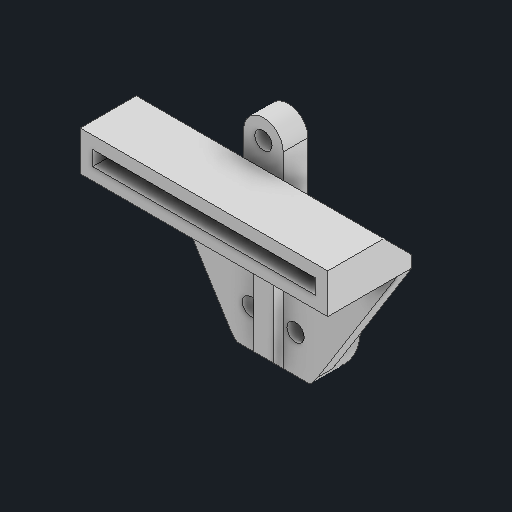
# Autodesk Inventor part: Lazercutlink
Saved by Autodesk Inventor 2026.1 (Build 301233000, 233)
## iProperties
Created: 2025-10-02
Part Number: Lazercutlink
Material: Generic
Document SubType Name: Modeling
Designer: Malthe Sennels
Density: 1 g/cm^3
Appearance: Default
Author: Malthe Sennels
Autodesk Inventor part; units mm, degrees
ref_plane "YZ Plane" through (0, 0, 0) normal (1, 0, 0) x (0, 1, 0)
ref_plane "XZ Plane" through (0, 0, 0) normal (0, 1, 0) x (-1, 0, 0)
ref_plane "XY Plane" through (0, 0, 0) normal (0, 0, 1) x (1, 0, 0)
sketch "Sketch1" plane through (0, 0, 0) normal (0, 0, 1) x (1, 0, 0)
  circle A0 centre (4.5, 0) radius 2.2 projected
  circle A1 centre (-4.5, 0) radius 2.2 projected
  circle A2 centre (0, 0) radius 10.6 projected
  circle A3 centre (4.5, 0) radius 1.75
  circle A4 centre (-4.5, 0) radius 1.75
  point P0 (0, 0)
  dimension "d0" = 3.5
  dimension "d1" = 3.5
  constraints: 2 centre point, 2 coincident
  measures "d0" diameter of A3
  measures "d1" diameter of A4
extrude "Extrusion1" add sketch "Sketch1" along normal blind 4 contours A0 | A1 | A2
sketch "Sketch2" plane through (0, 0, 0) normal (1, 0, 0) x (0, 1, 0)
  line L0 (10.6, 4) -> (-10.6, 4) projected
  line L1 (-10.6, 4) -> (-5.6, 9)
  line L2 (-5.6, 9) -> (16, 9)
  line L3 (16, 9) -> (20, 13)
  line L4 (20, 13) -> (20, 21)
  line L5 (20, 21) -> (28, 21)
  line L6 (28, 21) -> (28, 4)
  line L7 (28, 4) -> (10.6, 4)
  line L8 (28, 9.6863) -> (22.3137, 4)
  line L9 (28, 9.6863) -> (36.0416, 9.6863) construction
  point P0 (0, 0)
  point P1 (0, 4)
  dimension "d4" = 135
  dimension "d5" = 5
  dimension "d6" = 45
  dimension "d7" = 8
  dimension "d8" = 8
  dimension "d9" = 4
  dimension "d10" = 8
  dimension "d11" = 20
  constraints: 18 end point, 3 horizontal, 2 perpendicular, 2 point on line, 1 collinear, 1 equal length, 1 midpoint, 1 parallel
  measures "d4" angle of L8 L9
  measures "d5" distance between parallel lines of L7 L2
  measures "d6" angle of L0 L1
  measures "d7" distance between parallel lines of L3 L8
  measures "d8" distance between parallel lines of L6 L4
  measures "d9" distance from line of L2 L3.end
  measures "d10" distance from line of L3.end L5
  measures "d11" distance from line of point (0, 4) L4
extrude "Extrusion2" add sketch "Sketch2" along normal mid plane 4 contours L0 L1 L2 L3 L4 L5 L6 L8 L7
sketch "Sketch3" plane through (2, -10.6, 4) normal (0, 0, -1) x (-1, 0, 0)
  circle A0 centre (2, 10.6) radius 10.6 projected
  line L0 (4, 0) -> (2, 0) projected
  line L1 (2, 0) -> (0, 0) projected
  line L2 (0, 5) -> (0, 0) projected
  line L3 (4, 5) -> (0, 5) projected
  line L4 (4, 0) -> (4, 5) projected
  point P0 (2, 10.6)
  point P1 (0, 0.1904)
  point P2 (4, 0.1904)
extrude "Extrusion3" cut sketch "Sketch3" against normal through all contours A0 L1 L2 | L4 L0 A0
sketch "Sketch4" plane through (-2, 20, 21) normal (0, 0, 1) x (1, 0, 0)
  line L0 (4, 0) -> (0, 0) projected
  line L1 (4, 8) -> (4, 0) construction
  line L2 (0, 8) -> (4, 8) projected
  line L3 (0, 0) -> (0, 8) construction
  line L4 (0, 8) -> (4, 8) projected
  line L5 (2, 8) -> (2, 0)
  line L6 (0, 0) -> (4, 0) projected
  line L7 (-23, 8) -> (27, 8)
  line L8 (27, 8) -> (27, 0)
  line L9 (27, 0) -> (-23, 0)
  line L10 (-23, 0) -> (-23, 8)
  line L11 (-23, 8) -> (27, 0) construction
  line L12 (27, 8) -> (-23, 0) construction
  point P0 (2, -20)
  point P1 (2, 4)
  dimension "d16" = 50
  constraints: 14 end point, 5 midpoint, 2 parallel, 1 horizontal, 1 perpendicular, 1 point on line
  measures "d16" distance of L8.end L9.end
extrude "Extrusion4" add sketch "Sketch4" against normal up to surface surface through (0, 22.3137, 4) normal (0, 0.7071, -0.7071)
sketch "Sketch5" plane through (25, 20, 21) normal (1, 0, 0) x (0, 0, -1)
  line L0 (17, -9.5904) -> (17, 0) projected
  line L1 (19.3137, 0) -> (11.3137, 8) projected
  line L2 (0, 8) -> (11.3137, 8) projected
  line L3 (0, 0) -> (0, 8) projected
  line L4 (0, 0) -> (19.3137, 0) projected
  line L5 (17, 0) -> (17, 2.3137)
  line L6 (11.3137, 8) -> (19.3137, 0) projected
  point P0 (21, -20)
  constraints: 2 end point, 1 point on line, 1 vertical
extrude "Extrusion5" cut sketch "Sketch5" against normal through all contours L4 L5 L1
sketch "Sketch6" plane through (25, 20, 21) normal (0, 0, 1) x (1, 0, 0)
  line L0 (0, 0) -> (-50, 0) projected
  line L1 (0, 0) -> (0, 8) projected
  line L2 (-50, 8) -> (0, 8) projected
  line L3 (-50, 8) -> (-50, 0) projected
  line L4 (0, 0) -> (0, 8) projected
  line L5 (0, 4) -> (-50, 4) construction
  line L6 (-50, 8) -> (-50, 0) projected
  line L7 (-50, 8) -> (0, 8) projected
  line L8 (-25, 8) -> (-25, 0) construction
  line L9 (-27, 0) -> (-23, 0) projected
  line L10 (-17.5, 5.5) -> (-2.5, 5.5)
  line L11 (-2.5, 5.5) -> (-2.5, 2.5)
  line L12 (-2.5, 2.5) -> (-17.5, 2.5)
  line L13 (-17.5, 2.5) -> (-17.5, 5.5)
  line L14 (-17.5, 5.5) -> (-2.5, 2.5) construction
  line L15 (-2.5, 5.5) -> (-17.5, 2.5) construction
  line L16 (-32.5, 5.5) -> (-47.5, 5.5)
  line L17 (-47.5, 5.5) -> (-47.5, 2.5)
  line L18 (-47.5, 2.5) -> (-32.5, 2.5)
  line L19 (-32.5, 2.5) -> (-32.5, 5.5)
  point P0 (-25, -20)
  point P1 (-10, 4)
  dimension "d21" = 15
  dimension "d22" = 3
  dimension "d23" = 2.5
  constraints: 24 end point, 6 midpoint, 4 symmetric about line, 2 parallel, 1 horizontal, 1 perpendicular, 1 point on line
  measures "d21" distance of L11.end L12.end
  measures "d22" distance of L10.end L11.end
  measures "d23" distance between parallel lines of L1 L11
extrude "Extrusion6" cut sketch "Sketch6" against normal through all contours L10 L11 L12 L13 | L19 L18 L17 L16
sketch "Sketch7" plane through (25, 20, 21) normal (0, 0, 1) x (1, 0, 0)
  line L0 (-17.5, 2.5) -> (-17.5, 5.5) projected
  line L1 (-32.5, 5.5) -> (-32.5, 2.5) projected
  line L2 (-17.5, 5.5) -> (-32.5, 5.5)
  line L3 (-32.5, 5.5) -> (-32.5, 2.5)
  line L4 (-32.5, 2.5) -> (-17.5, 2.5)
  line L5 (-17.5, 2.5) -> (-17.5, 5.5)
  point P0 (-25, -20)
  constraints: 8 end point, 2 parallel, 1 horizontal, 1 perpendicular
extrude "Extrusion7" cut sketch "Sketch7" against normal blind 6
sketch "Sketch8" plane through (0, 0, 4) normal (0, 0, 1) x (1, 0, 0)
  circle A0 centre (4.5, 0) radius 1.75 projected
  line L0 (2, 10.4096) -> (2, -10.4096) projected
  line L1 (2, 20) -> (25, 20) projected
  line L2 (25, 20) -> (8.9888, -5.618)
  arc A1 (2, -10.4096) -> (2, 10.4096) centre (0, 0) ccw projected
  line L3 (2, 5.8415) -> (10.849, 20)
  arc A2 (-2, -10.4096) -> (2, -10.4096) centre (0, 0) ccw projected
  line L4 (0, -10.6) -> (0, 30.6147)
  line L5 (-25, 20) -> (-8.9888, -5.618)
  line L6 (-2, 5.8415) -> (-10.849, 20)
  arc A3 (-2, 10.4096) -> (-2, -10.4096) centre (0, 0) ccw projected
  line L7 (-13.7579, -10.035) -> (-3.7579, -10.035) projected
  line L8 (-25, 20) -> (-2, 20) projected
  point P0 (0, 0)
  dimension "d29" = 12
  constraints: 10 end point, 4 symmetric about line, 2 point on line, 1 parallel, 1 point on circle, 1 tangent, 1 vertical
  measures "d29" distance between parallel lines of L2 L3
extrude "Extrusion8" add sketch "Sketch8" along normal blind 3 contours L3 A1 L0 | L3 L1 L2 A1 picked at (5.0326, 4.687)
sketch "Sketch9" plane through (2, -10.4096, 7) normal (-1, 0, 0) x (0, 0, 1)
  line L0 (0, 2.8096) -> (-2.8096, 0) projected
  line L1 (-2.8096, 0) -> (0, 0) projected
  line L2 (0, 2.8096) -> (0, 0) projected
  point P0 (-7, 10.4096)
extrude "Extrusion9" cut sketch "Sketch9" against normal through all
mirror "Mirror1" about plane through (0, 0, 0) normal (1, 0, 0) of "Extrusion8", "Extrusion9"
sketch "Sketch10" plane through (0, 0, 4) normal (0, 0, -1) x (-1, 0, 0)
  circle A0 centre (0, 32.3137) radius 1.75
  circle A1 centre (0, 32.3137) radius 4
  line L0 (-4, 32.3137) -> (-4, 22.3137)
  line L1 (-25, 22.3137) -> (25, 22.3137) projected
  line L2 (0, 22.3137) -> (0, 32.3137) construction
  line L3 (4, 32.3137) -> (4, 22.3137)
  point P0 (0, 0)
  dimension "d36" = 8
  dimension "d34" = 3.5
  dimension "d35" = 10
  constraints: 6 end point, 3 vertical, 2 symmetric about line, 1 centre point, 1 coincident, 1 midpoint, 1 point on line, 3 other
  measures "d34" diameter of A0
  measures "d35" distance from line of L1 A0.centre
extrude "Extrusion10" add sketch "Sketch10" against normal blind 5
body "Solid1"
